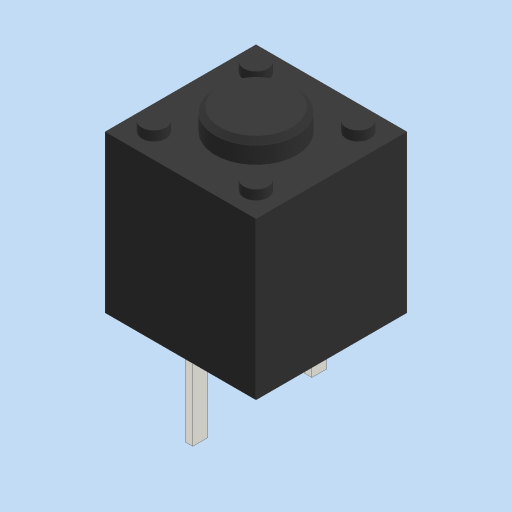
# Autodesk Inventor part: 6mm_switch
Saved by Autodesk Inventor 2024 (Build 280153000, 153)
## iProperties
Created: 2025-05-06
Part Number: 6mm_switch
Material: Generic
Document SubType Name: Modeling
Designer: XxPan
Density: 1 g/cm^3
Appearance: Default
Author: XxPan
Autodesk Inventor part; units mm, degrees
ref_plane "YZ Plane" through (0, 0, 0) normal (1, 0, 0) x (0, 1, 0)
ref_plane "XZ Plane" through (0, 0, 0) normal (0, 1, 0) x (-1, 0, 0)
ref_plane "XY Plane" through (0, 0, 0) normal (0, 0, 1) x (1, 0, 0)
sketch "Sketch1" plane through (0, 0, 0) normal (0, 1, 0) x (-1, 0, 0)
  line L0 (3.1, 3.1) -> (-3.1, 3.1)
  line L1 (-3.1, 3.1) -> (-3.1, -3.1)
  line L2 (-3.1, -3.1) -> (3.1, -3.1)
  line L3 (3.1, -3.1) -> (3.1, 3.1)
  line L4 (4.34, 0) -> (-4.34, 0) construction
  line L5 (0, -4.34) -> (0, 4.34) construction
  point P0 (0, 0)
  dimension "d0" = 6.2
  dimension "d1" = 6.2
  constraints: 8 end point, 2 parallel, 1 horizontal, 1 perpendicular, 2 other
  measures "d0" distance of L2.end L1.end
  measures "d1" distance of L1.end L0.end
extrude "Extrusion1" add sketch "Sketch1" along normal blind 6.45
sketch "Sketch2" plane through (0, 6.45, 0) normal (0, 1, 0) x (1, 0, 0)
  circle A0 centre (-2.1, -2.1) radius 0.5
  circle A1 centre (-2.1, 2.1) radius 0.5
  circle A2 centre (2.1, 2.1) radius 0.5
  circle A3 centre (2.1, -2.1) radius 0.5
  line L0 (-3.1, -3.1) -> (3.1, -3.1) projected
  line L1 (-3.1, 3.1) -> (-3.1, -3.1) projected
  line L2 (3.1, 3.1) -> (-3.1, 3.1) projected
  line L3 (3.1, -3.1) -> (3.1, 3.1) projected
  point P0 (0, 0)
  dimension "d4" = 1
  dimension "d5" = 1
  dimension "d6" = 1
  dimension "d7" = 1
  dimension "d8" = 1
  dimension "d9" = 1
  dimension "d10" = 1
  dimension "d11" = 1
  constraints: 4 centre point, 2 horizontal alignment, 2 vertical alignment
  measures "d4" diameter of A0
  measures "d5" diameter of A1
  measures "d6" diameter of A2
  measures "d7" diameter of A3
  measures "d8" distance from line of L0 A0.centre
  measures "d9" distance from line of L1 A0.centre
  measures "d10" distance from line of L2 A1.centre
  measures "d11" distance from line of L3 A3.centre
extrude "Extrusion2" add sketch "Sketch2" along normal blind 0.4 contours A0 | A1 | A2 | A3
sketch "Sketch3" plane through (0, 6.45, 0) normal (0, 1, 0) x (1, 0, 0)
  circle A0 centre (0, 0) radius 1.675
  dimension "d14" = 3.35
  constraints: 1 centre point, 1 coincident
  measures "d14" diameter of A0
extrude "Extrusion3" add sketch "Sketch3" along normal blind 0.9
chamfer "Chamfer1" distance 0.2 angle 45 1 edges at (-1.675, 7.35, 0)
sketch "Sketch4" plane through (0, 0, 0) normal (1, 0, 0) x (0, 1, 0)
  line L0 (0, 3.1) -> (0, -3.1) projected
  line L1 (0, 2.75) -> (-3.3, 2.75)
  line L2 (-3.3, 2.75) -> (-3.3, 2.15)
  line L3 (-3.3, 2.15) -> (0, 2.15)
  line L4 (0, -2.15) -> (-3.3, -2.15)
  line L5 (-3.3, -2.15) -> (-3.3, -2.75)
  line L6 (-3.3, -2.75) -> (0, -2.75)
  line L7 (-3.96, 0) -> (0.66, 0) projected
  point P0 (0, 0)
  dimension "d20" = 5.5
  dimension "d21" = 0.6
  dimension "d22" = 0.6
  dimension "d23" = 3.3
  constraints: 12 end point, 6 point on line, 3 perpendicular, 1 horizontal, 1 parallel, 1 other
  measures "d20" distance between parallel lines of L6 L1
  measures "d21" distance of L1.end L2.end
  measures "d22" distance of L4.end L5.end
  measures "d23" distance between parallel lines of L0 L2
extrude "Extrusion4" add sketch "Sketch4" along normal mid plane 0.3
body "Solid1"
